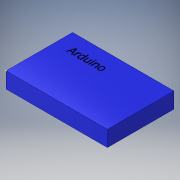
# Autodesk Inventor part: Arduino
Saved by Autodesk Inventor 2019.4 (Build 234330000, 330)
## iProperties
Created: 2019-06-13
Part Number: Arduino
Material: Generic
Document SubType Name: Modeling
Designer: abdel
Density: 1 g/cm^3
Appearance: Blue - Wall Paint - Glossy
Author: abdel
Autodesk Inventor part; units mm, degrees
ref_plane "YZ Plane" through (0, 0, 0) normal (1, 0, 0) x (0, 1, 0)
ref_plane "XZ Plane" through (0, 0, 0) normal (0, 1, 0) x (-1, 0, 0)
ref_plane "XY Plane" through (0, 0, 0) normal (0, 0, 1) x (1, 0, 0)
sketch "Sketch1" plane through (0, 0, 0) normal (0, 1, 0) x (-1, 0, 0)
  line L0 (0, 0) -> (-81.28, 0)
  line L1 (-81.28, 0) -> (-81.28, -53.34)
  line L2 (-81.28, -53.34) -> (0, -53.34)
  line L3 (0, -53.34) -> (0, 0)
  dimension "d0" = 81.28
  dimension "d1" = 53.34
  constraints: 8 end point, 2 parallel, 1 horizontal, 1 perpendicular
  measures "d0" distance of L2.end L1.end
  measures "d1" distance of L1.end L0.end
extrude "Extrusion1" add sketch "Sketch1" along normal blind 12.7
sketch "Sketch2" plane through (0, 12.7, 0) normal (0, 1, 0) x (1, 0, 0)
  line L0 (10.2876, 43.9262) -> (61.9475, 43.9262) construction
  line L1 (61.9475, 43.9262) -> (61.9475, 11.4305) construction
  line L2 (61.9475, 11.4305) -> (10.2876, 11.4305) construction
  line L3 (10.2876, 11.4305) -> (10.2876, 43.9262) construction
  point P0 (0, 0)
  constraints: 2 other
body "Solid1"
